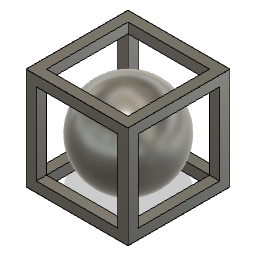
cube_sphere (Autodesk Fusion 360 design; units mm, degrees)
Autodesk Fusion 360 part; units mm, degrees
box "BoxPrimitive1" add length 50 width 50 height 50 placed x (0, 0, 1) y (1, 0, 0) z (0, 1, 0) at (0, 0, 0) makes body 1
sketch "Sketch4" plane through (0, 50, 0) normal (0, 1, 0) x (-1, 0, 0)
  line L0 (0, 50) -> (-50, 50)
  line L1 (-50, 50) -> (-50, 0)
  line L2 (-50, 0) -> (0, 0)
  line L3 (0, 0) -> (0, 50)
  line L4 (-5, 5) -> (-45, 5)
  line L5 (-45, 5) -> (-45, 45)
  line L6 (-45, 45) -> (-5, 45)
  line L7 (-5, 45) -> (-5, 5)
  constraint horizontal L4
  constraint vertical L5
  constraint horizontal L6
  constraint vertical L7
extrude "Extrude1" cut sketch "Sketch4" against normal blind 55 contours L4 L5 L6 L7 bodies 1
sketch "Sketch5" plane through (50, 0, 0) normal (1, 0, 0) x (0, 0, -1)
  line L0 (-50, 50) -> (-50, 0)
  line L1 (-50, 0) -> (0, 0)
  line L2 (0, 0) -> (0, 50)
  line L3 (0, 50) -> (-50, 50)
  line L4 (-45, 45) -> (-5, 45)
  line L5 (-5, 45) -> (-5, 5)
  line L6 (-5, 5) -> (-45, 5)
  line L7 (-45, 5) -> (-45, 45)
  constraint horizontal L4
  constraint vertical L5
  constraint horizontal L6
  constraint vertical L7
extrude "Extrude2" cut sketch "Sketch5" against normal blind 55 contours L4 L5 L6 L7 bodies 1
sketch "Sketch6" plane through (0, 0, 50) normal (0, 0, 1) x (1, 0, 0)
  line L0 (0, 50) -> (0, 0)
  line L1 (0, 0) -> (50, 0)
  line L2 (50, 0) -> (50, 50)
  line L3 (50, 50) -> (0, 50)
  line L4 (5, 45) -> (45, 45)
  line L5 (45, 45) -> (45, 5)
  line L6 (45, 5) -> (5, 5)
  line L7 (5, 5) -> (5, 45)
  constraint horizontal L4
  constraint vertical L5
  constraint horizontal L6
  constraint vertical L7
extrude "Extrude3" cut sketch "Sketch6" against normal blind 55 contours L4 L5 L6 L7 bodies 1
sphere "SpherePrimitive1" add diameter 45 placed x (1, 0, 0) y (0, 0, -1) z (0, 1, 0) at (12.3413, 0, 127.4383) separate body makes body 2
move_body "MoveFace1" bodies 2 to x (1, 0, 0) y (0, 1, 0) z (0, 0, 1) at (12.5261, 0, -102.6717) on bodies 2
move_body "MoveFace2" bodies 2 to x (1, 0, 0) y (0, 1, 0) z (0, 0, 1) at (0, 20, 0) on bodies 2
move_body "Align1" bodies 1 to x (1, 0, 0) y (0, 1, 0) z (0, 0, 1) at (0, 15, 0)
move_body "Move1" bodies 1 to x (1, 0, 0) y (0, 1, 0) z (0, 0, 1) at (0, -15, 0)
move_body "MoveFace3" bodies 2 to x (1, 0, 0) y (0, 1, 0) z (0, 0, 1) at (0, 2.5, 0) on bodies 2
